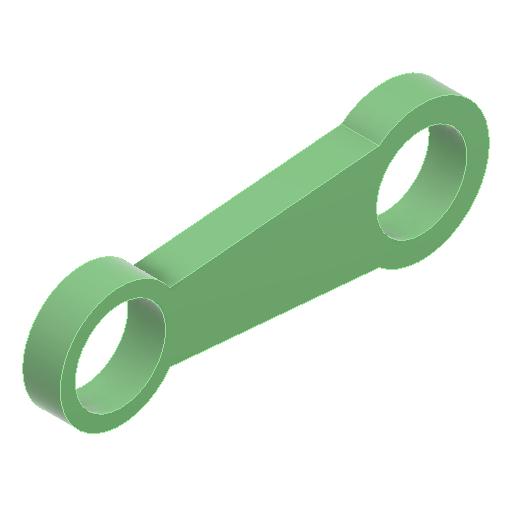
# Autodesk Inventor part: Link_OD
Saved by Autodesk Inventor 2026.2 (Build 302298000, 298)
## iProperties
Created: 2025-12-27
Part Number: Link_OD
Material: ABS 塑膠
Document SubType Name: Modeling
Designer: Hsiangyu
Density: 1.06 g/cm^3
Appearance: 平滑 - 深森林綠
Author: Hsiangyu
Autodesk Inventor part; units mm, degrees
ref_plane "YZ Plane" through (0, 0, 0) normal (1, 0, 0) x (0, 1, 0)
ref_plane "XZ Plane" through (0, 0, 0) normal (0, 1, 0) x (-1, 0, 0)
ref_plane "XY Plane" through (0, 0, 0) normal (0, 0, 1) x (1, 0, 0)
sketch "草圖1" plane through (0, 0, 0) normal (1, 0, 0) x (0, 1, 0)
  line L0 (0, 0) -> (0, 40)
  circle A0 centre (0, 40) radius 6
  circle A1 centre (0, 0) radius 6
  circle A2 centre (0, 40) radius 8
  circle A3 centre (0, 0) radius 9
  line L1 (7, 5.6569) -> (4.5698, 33.4337)
  line L2 (-4.5698, 33.4337) -> (-7, 5.6569)
  dimension "d0" = 40
  dimension "d1" = 12
  dimension "d2" = 16
  dimension "d3" = 18
  dimension "d4" = 5
  dimension "d5" = 5
  dimension "d6" = 7
  dimension "d7" = 7
  constraints: 6 end point, 4 centre point, 4 coincident, 4 point on circle, 1 equal radius, 1 vertical
  measures "d0" distance of L0.start L0.end
  measures "d1" diameter of A0
  measures "d2" diameter of A2
  measures "d3" diameter of A3
  measures "d4" angle of L0 L2
  measures "d5" angle of L0 L1
  measures "d6" distance from line of L0 L1.start
  measures "d7" horizontal distance of L0.start L2.end
extrude "擠出1" add sketch "草圖1" along normal mid plane 5
equation "\"d5\" = d4"
equation "\"d7\" = d6"
